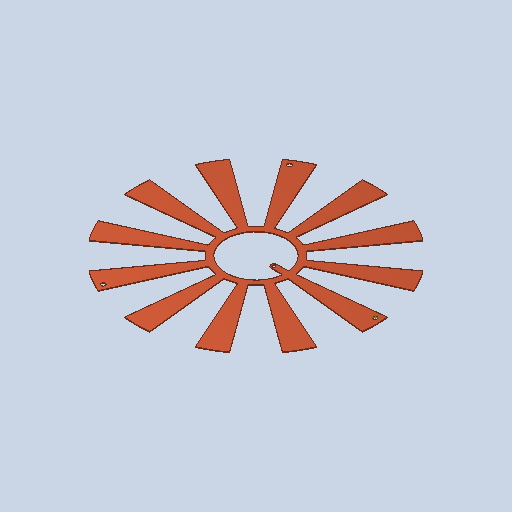
# Autodesk Inventor part: torsosc-electrode-pcb-cu
Saved by Autodesk Inventor 2026 (Build 300175050, 175E)
## iProperties
Created: 2021-01-06
Part Number: torsosc-electrode-pcb-cu
Material: Copper
Document SubType Name: Modeling
Designer: schanen
Density: 8.94 g/cm^3
Appearance: Copper - Satin
Author: schanen
Autodesk Inventor part; units mm, degrees
ref_plane "YZ Plane" through (0, 0, 0) normal (1, 0, 0) x (0, 1, 0)
ref_plane "XZ Plane" through (0, 0, 0) normal (0, 1, 0) x (-1, 0, 0)
ref_plane "XY Plane" through (0, 0, 0) normal (0, 0, 1) x (1, 0, 0)
sketch "Sketch4" plane through (0, 0, 0) normal (0, 1, 0) x (-1, 0, 0)
  circle A0 centre (0, 0) radius 6 construction
  circle A1 centre (0, 0) radius 20 construction
  line L0 (0, 0) -> (-19.8904, -2.0906) construction
  line L1 (0, 0) -> (-19.8904, 2.0906) construction
  line L2 (28, 0) -> (-28, 0) projected
  arc A2 (-19.8904, 2.0906) -> (-19.8904, -2.0906) centre (0, 0) ccw
  line L3 (-19.8904, 2.0906) -> (-5.9671, 0.6272)
  line L4 (-19.8904, -2.0906) -> (-5.9671, -0.6272)
  arc A3 (-5.9671, 0.6272) -> (-5.9671, -0.6272) centre (0, 0) ccw
  dimension "d38" = 12
  dimension "d39" = 40
  dimension "d41" = 6
  dimension "d42" = 6
  constraints: 8 end point, 8 point on circle, 4 centre point, 3 coincident, 2 point on line
  measures "d38" diameter of A0
  measures "d39" diameter of A1
  measures "d41" angle of L2 L0
  measures "d42" angle of L2 L1
extrude "Extrusion5" add sketch "Sketch4" along normal blind 0.1
pattern_circular "Circular Pattern1" count 12 over 360 about axis through (0, -10, 0) along (0, 1, 0) of "Extrusion5"
sketch "Sketch5" plane through (0, 0.1, 0) normal (0, 1, 0) x (1, 0, 0)
  arc A0 (5.4813, 2.4404) -> (4.8541, 3.5267) centre (0, 0) ccw projected
  arc A1 (5.9671, -0.6272) -> (5.9671, 0.6272) centre (0, 0) ccw projected
  circle A2 centre (0, 0) radius 6
  circle A3 centre (0, 0) radius 5
  point P0 (4.8541, 3.5267)
  point P1 (5.9671, 0.6272)
  point P2 (5.4813, 2.4404)
  dimension "d48" = 1
  constraints: 2 centre point, 2 coincident, 1 concentric
  measures "d48" radial gap between concentric circles of A2 A3
extrude "Extrusion6" add sketch "Sketch5" against normal blind 0.1
sketch "Sketch7" plane through (0, 0.1, 0) normal (0, 1, 0) x (1, 0, 0)
  circle A0 centre (0, 0) radius 19 construction
  point P0 (18.974, 0.9944)
  point P1 (19, 0)
  dimension "d55" = 38
  dimension "d56" = 3
  constraints: 2 horizontal alignment, 1 coincident, 2 other
hole "Hole1" at (18.974, 0.1, -0.9944) direction (0, -1, 0) diameter 0.7 end through all
pattern_circular "Circular Pattern2" count 3 over 360 about axis through (0, -10, 0) along (0, 1, 0) of "Hole1"
sketch "Sketch8" plane through (0, 0.1, 0) normal (0, 1, 0) x (1, 0, 0)
  circle A0 centre (0, 0) radius 2.5 construction
  circle A1 centre (0, 0) radius 5 projected
  line L0 (5, 0) -> (3, 0)
  line L1 (3, 0) -> (3, 0.5)
  line L2 (3, 0.5) -> (5, 0.5)
  line L3 (5, 0.5) -> (5, 0)
  line L4 (5, 0) -> (3, 0)
  line L5 (3, 0) -> (3, -0.5)
  line L6 (3, -0.5) -> (5, -0.5)
  line L7 (5, -0.5) -> (5, 0)
  circle A2 centre (3, 0) radius 0.5
  circle A3 centre (3, 0) radius 0.25
  point P0 (4.9749, -0.5)
  point P1 (4.9749, 0.5)
  dimension "d67" = 5
  dimension "d68" = 2
  dimension "d69" = 0.5
  dimension "d70" = 0.5
  dimension "d71" = 0.5
  constraints: 16 end point, 4 parallel, 3 coincident, 2 centre point, 2 horizontal, 2 perpendicular, 5 other
  measures "d67" diameter of A0
  measures "d68" distance of L1.end L2.end
  measures "d69" distance of L0.end L1.end
  measures "d70" distance of L5.end L4.end
  measures "d71" diameter of A3
extrude "Extrusion8" add sketch "Sketch8" against normal blind 0.1 contours L0 A2 L2 A1 | A1 L6 A2 L0 | A2 L5 A3 L0 | L0 A3 L1 A2 | L1 A3 L5 A2
fillet "Fillet5" radius 0.2 2 edges at (5.9671, 0.05, 0.6272) (5.9671, 0.05, -0.6272)
pattern_circular "Circular Pattern3" count 12 over 360 about axis through (0, 0.1, 0) along (0, -1, 0) of "Fillet5"
fillet "Fillet6" radius 0.2 2 edges at (4.9749, 0.05, -0.5) (4.9749, 0.05, 0.5)
equation "\"d42\" = d41"
body "Solid2"
